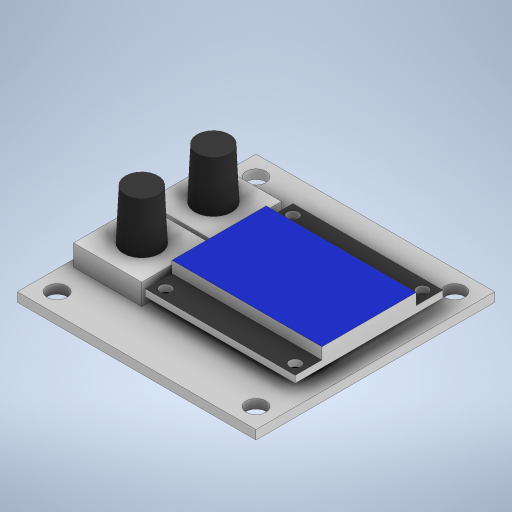
# Autodesk Inventor part: display_buttons
Saved by Autodesk Inventor 2023 (Build 270158000, 158)
## iProperties
Created: 2023-05-18
Part Number: display_buttons
Material: Generic
Document SubType Name: Modeling
Designer: mark
Density: 1 g/cm^3
Appearance: Default
Author: mark
Autodesk Inventor part; units mm, degrees
ref_plane "YZ Plane" through (0, 0, 0) normal (1, 0, 0) x (0, 1, 0)
ref_plane "XZ Plane" through (0, 0, 0) normal (0, 1, 0) x (-1, 0, 0)
ref_plane "XY Plane" through (0, 0, 0) normal (0, 0, 1) x (1, 0, 0)
sketch "Sketch1" plane through (0, 0, 0) normal (0, 1, 0) x (-1, 0, 0)
  line L0 (64.0448, -68.929) -> (37.6448, -68.929)
  line L1 (37.6448, -68.929) -> (37.6448, -42.929)
  line L2 (37.6448, -42.929) -> (64.0448, -42.929)
  line L3 (64.0448, -42.929) -> (64.0448, -68.929)
  point P0 (0, 0)
  dimension "d0" = 26.4
  dimension "d1" = 26
  constraints: 8 end point, 2 parallel, 1 horizontal, 1 perpendicular
  measures "d0" distance of L1.end L2.end
  measures "d1" distance of L0.end L1.end
extrude "Extrusion1" add sketch "Sketch1" along normal blind 1.2
sketch "Sketch2" plane through (0, 1.2, 0) normal (0, 1, 0) x (1, 0, 0)
  line L0 (-64.0448, 68.929) -> (-64.0448, 42.929) projected
  line L1 (-37.6448, 42.929) -> (-37.6448, 68.929) projected
  line L2 (-64.0448, 64.229) -> (-37.6448, 64.229)
  line L3 (-37.6448, 64.229) -> (-37.6448, 47.629)
  line L4 (-37.6448, 47.629) -> (-64.0448, 47.629)
  line L5 (-64.0448, 47.629) -> (-64.0448, 64.229)
  line L6 (-37.6448, 68.929) -> (-64.0448, 68.929) projected
  point P0 (0, 0)
  dimension "d4" = 4.7
  dimension "d5" = 16.6
  constraints: 8 end point, 2 parallel, 2 point on line, 1 horizontal, 1 perpendicular
  measures "d4" distance between parallel lines of L2 L6
  measures "d5" distance between parallel lines of L2 L4
extrude "Extrusion2" add sketch "Sketch2" along normal blind 2 contours L2 L1 L4 L0
sketch "Sketch3" plane through (0, 1.2, 0) normal (0, 1, 0) x (1, 0, 0)
  circle A0 centre (-62.2448, 67.129) radius 1
  circle A1 centre (-39.4448, 67.129) radius 1
  circle A2 centre (-39.4448, 44.729) radius 1
  circle A3 centre (-62.2448, 44.729) radius 1
  line L0 (-64.0448, 68.929) -> (-64.0448, 64.229) projected
  line L1 (-37.6448, 68.929) -> (-64.0448, 68.929) projected
  line L2 (-37.6448, 64.229) -> (-37.6448, 68.929) projected
  line L3 (-37.6448, 42.929) -> (-37.6448, 47.629) projected
  line L4 (-64.0448, 42.929) -> (-37.6448, 42.929) projected
  line L5 (-64.0448, 47.629) -> (-64.0448, 42.929) projected
  point P0 (0, 0)
  point P1 (-64.0448, 45.279)
  dimension "d8" = 2
  dimension "d9" = 2
  dimension "d10" = 2
  dimension "d11" = 2
  dimension "d12" = 1.8
  dimension "d13" = 1.8
  dimension "d14" = 1.8
  dimension "d15" = 1.8
  dimension "d16" = 1.8
  dimension "d17" = 1.8
  dimension "d18" = 1.8
  dimension "d19" = 1.8
  constraints: 4 centre point, 1 midpoint
  measures "d8" diameter of A0
  measures "d9" diameter of A1
  measures "d10" diameter of A2
  measures "d11" diameter of A3
  measures "d12" distance from line of L0 A0.centre
  measures "d13" distance from line of L1 A0.centre
  measures "d14" distance from line of L1 A1.centre
  measures "d15" distance from line of L2 A1.centre
  measures "d16" distance from line of L3 A2.centre
  measures "d17" distance from line of L4 A2.centre
  measures "d18" distance from line of L4 A3.centre
  measures "d19" horizontal distance of point (-64.045, 45.279) A3.centre
extrude "Extrusion3" cut sketch "Sketch3" against normal through all
sketch "Sketch4" plane through (0, 0, 0) normal (0, -1, 0) x (1, 0, 0)
  line L0 (-45.8948, -68.929) -> (-55.8948, -68.929)
  line L1 (-55.8948, -68.929) -> (-55.8948, -66.429)
  line L2 (-55.8948, -66.429) -> (-45.8948, -66.429)
  line L3 (-45.8948, -66.429) -> (-45.8948, -68.929)
  line L4 (-37.6448, -68.929) -> (-64.0448, -68.929) projected
  line L5 (-37.6448, -42.929) -> (-37.6448, -68.929) projected
  point P0 (0, 0)
  dimension "d22" = 10
  dimension "d23" = 2.5
  dimension "d24" = 0
  dimension "d25" = 8.25
  constraints: 8 end point, 2 parallel, 1 horizontal, 1 perpendicular
  measures "d22" distance of L1.end L2.end
  measures "d23" distance of L0.end L1.end
  measures "d24" distance between parallel lines of L4 L0
  measures "d25" distance between parallel lines of L5 L3
extrude "Extrusion4" add sketch "Sketch4" along normal blind 2.5
sketch "Sketch5" plane through (0, -2.5, 0) normal (0, -1, 0) x (1, 0, 0)
  line L0 (-65.3448, -68.229) -> (-77.3448, -68.229)
  line L1 (-77.3448, -68.229) -> (-77.3448, -56.229)
  line L2 (-77.3448, -56.229) -> (-65.3448, -56.229)
  line L3 (-65.3448, -56.229) -> (-65.3448, -68.229)
  line L4 (-65.3448, -55.629) -> (-77.3448, -55.629)
  line L5 (-77.3448, -55.629) -> (-77.3448, -43.629)
  line L6 (-77.3448, -43.629) -> (-65.3448, -43.629)
  line L7 (-65.3448, -43.629) -> (-65.3448, -55.629)
  line L8 (-55.8948, -68.929) -> (-64.0448, -68.929) projected
  line L9 (-64.0448, -68.929) -> (-64.0448, -42.929) projected
  line L10 (-64.0448, -42.929) -> (-37.6448, -42.929) projected
  point P0 (0, 0)
  dimension "d28" = 12
  dimension "d29" = 12
  dimension "d30" = 12
  dimension "d31" = 12
  dimension "d32" = 0.7
  dimension "d33" = 1.3
  dimension "d34" = 0.7
  constraints: 16 end point, 4 parallel, 2 horizontal, 2 perpendicular, 1 point on line
  measures "d28" distance of L1.end L2.end
  measures "d29" distance of L0.end L1.end
  measures "d30" distance of L5.end L6.end
  measures "d31" distance of L4.end L5.end
  measures "d32" distance between parallel lines of L8 L0
  measures "d33" distance between parallel lines of L9 L3
  measures "d34" distance between parallel lines of L10 L6
extrude "Extrusion5" add sketch "Sketch5" against normal blind 3.7
sketch "Sketch7" plane through (0, 1.2, 0) normal (0, 1, 0) x (1, 0, 0)
  circle A0 centre (-71.3448, 62.229) radius 3.25
  circle A1 centre (-71.3448, 49.629) radius 3.25
  line L0 (-65.3448, 68.229) -> (-77.3448, 68.229) projected
  line L1 (-77.3448, 68.229) -> (-77.3448, 43.629) projected
  line L2 (-65.3448, 55.629) -> (-77.3448, 55.629) projected
  line L3 (-77.3448, 55.629) -> (-77.3448, 43.629) projected
  point P0 (0, 0)
  point P1 (-77.3448, 56.229)
  dimension "d47" = 6.5
  dimension "d48" = 6.5
  dimension "d49" = 6
  dimension "d50" = 6
  dimension "d51" = 6
  dimension "d52" = 6
  constraints: 2 centre point
  measures "d47" diameter of A0
  measures "d48" diameter of A1
  measures "d49" distance from line of L0 A0.centre
  measures "d50" distance from line of L1 A0.centre
  measures "d51" distance from line of L2 A1.centre
  measures "d52" distance from line of L3 A1.centre
extrude "Extrusion7" add sketch "Sketch7" along normal blind 8.8
draft "FaceDraft3" angle 2.5 pull direction (0, 1, 0) faces at (-68.1053, 7.0667, -61.9675) fixed edges at (-74.5948, 1.2, -62.229)
draft "FaceDraft4" angle 2.5 pull direction (0, 1, 0) faces at (-68.1053, 7.0667, -49.3675) fixed edges at (-74.5948, 1.2, -49.629)
sketch "Sketch8" plane through (0, -2.5, 0) normal (0, -1, 0) x (1, 0, 0)
  line L0 (-78.5448, -34.929) -> (-36.5448, -34.929)
  line L1 (-36.5448, -34.929) -> (-36.5448, -76.929)
  line L2 (-36.5448, -76.929) -> (-78.5448, -76.929)
  line L3 (-78.5448, -76.929) -> (-78.5448, -34.929)
  line L4 (-64.0448, -42.929) -> (-37.6448, -42.929) projected
  line L5 (-37.6448, -42.929) -> (-37.6448, -68.929) projected
  circle A0 centre (-75.0448, -73.429) radius 1.75
  circle A1 centre (-40.0448, -73.429) radius 1.75
  circle A2 centre (-75.0448, -38.429) radius 1.75
  circle A3 centre (-40.0448, -38.429) radius 1.75
  line L6 (-37.6448, -47.629) -> (-37.6448, -64.229) projected
  point P0 (0, 0)
  point P1 (-37.6448, -55.929)
  dimension "d57" = 42
  dimension "d58" = 42
  dimension "d59" = 8
  dimension "d63" = 3.5
  dimension "d64" = 3.5
  dimension "d65" = 3.5
  dimension "d66" = 3.5
  dimension "d67" = 3.5
  dimension "d68" = 3.5
  dimension "d69" = 3.5
  dimension "d70" = 3.5
  dimension "d71" = 3.5
  dimension "d72" = 3.5
  dimension "d73" = 3.5
  dimension "d74" = 3.5
  dimension "d75" = 1.1
  constraints: 8 end point, 4 centre point, 2 parallel, 1 horizontal, 1 midpoint, 1 perpendicular
  measures "d57" distance of L0.start L0.end
  measures "d58" distance of L0.end L1.end
  measures "d59" distance between parallel lines of L4 L0
  measures "d63" diameter of A0
  measures "d64" diameter of A1
  measures "d65" diameter of A2
  measures "d66" diameter of A3
  measures "d67" distance from line of L2 A0.centre
  measures "d68" distance from line of L3 A0.centre
  measures "d69" distance from line of L1 A1.centre
  measures "d70" distance from line of L2 A1.centre
  measures "d71" distance from line of L1 A3.centre
  measures "d72" distance from line of L0 A3.centre
  measures "d73" distance from line of L0 A2.centre
  measures "d74" distance from line of L3 A2.centre
  measures "d75" distance from line of point (-37.645, -55.929) L1
extrude "Extrusion8" add sketch "Sketch8" along normal blind 1.6
equation "\"d14\" = d13"
equation "\"d15\" = d14"
equation "\"d16\" = d14"
equation "\"d17\" = d15"
equation "\"d18\" = d12"
equation "\"d51\" = d49"
equation "\"d52\" = d50"
equation "\"d64\" = d63"
equation "\"d65\" = d63"
equation "\"d66\" = d63"
equation "\"d68\" = d67"
equation "\"d69\" = d68"
equation "\"d70\" = d68"
equation "\"d71\" = d69"
equation "\"d72\" = d70"
equation "\"d73\" = d67"
equation "\"d74\" = d68"
body "Solid1"
